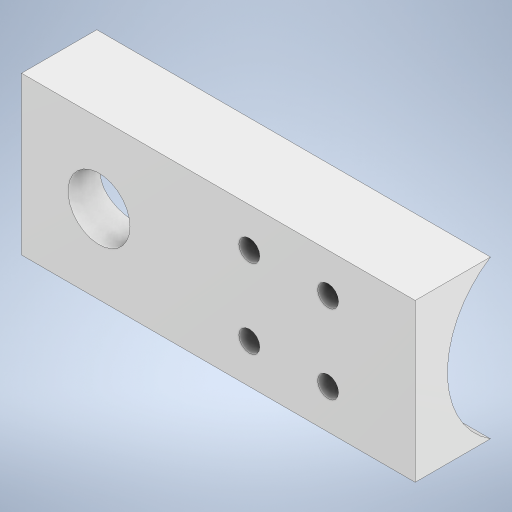
# Autodesk Inventor part: Motor Mount
Saved by Autodesk Inventor 2023 (Build 270158030, 158C)
## iProperties
Created: 2022-10-03
Part Number: Motor Mount
Material: ABS Plastic
Document SubType Name: Modeling
Designer: cjj5381
Density: 1.06 g/cm^3
Appearance: Smooth - White
Author: cjj5381
Autodesk Inventor part; units mm, degrees
ref_plane "YZ Plane" through (0, 0, 0) normal (1, 0, 0) x (0, 1, 0)
ref_plane "XZ Plane" through (0, 0, 0) normal (0, 1, 0) x (-1, 0, 0)
ref_plane "XY Plane" through (0, 0, 0) normal (0, 0, 1) x (1, 0, 0)
sketch "Sketch1" plane through (0, 0, 0) normal (1, 0, 0) x (0, 1, 0)
  arc A0 (25.4, -19.293) -> (-25.4, -19.293) centre (0, -35.56) ccw
  line L0 (0, 0) -> (0, -134.2841)
  line L1 (-25.4, 0) -> (-25.4, -19.293)
  line L2 (25.4, -19.293) -> (25.4, 0)
  line L3 (25.4, 0) -> (25.4, 5)
  line L4 (25.4, 5) -> (-25.4, 5)
  line L5 (-25.4, 5) -> (-25.4, 0)
  dimension "d0" = 60.325
  dimension "d3" = 50.8
  dimension "d38" = 5
  constraints: 12 end point, 2 perpendicular, 2 point on circle, 2 vertical, 1 centre point, 1 parallel, 1 point on line, 1 other
  measures "d0" diameter of A0
  measures "d3" distance between parallel lines of L1 L2
  measures "d38" distance from line of L0.start L4
extrude "Extrusion1" add sketch "Sketch1" along normal blind 127
sketch "Sketch4" plane through (0, 25.4, 5) normal (0, 0, 1) x (1, 0, 0)
  circle A0 centre (25, -25.4) radius 10
  line L0 (0, 0) -> (127, 0) projected
  line L1 (0, 0) -> (0, -50.8) projected
  dimension "d20" = 20
  dimension "d39" = 25.4
  dimension "d40" = 25
  constraints: 1 centre point, 1 coincident
  measures "d20" diameter of A0
  measures "d39" distance from line of point (25, -25.4) L0
  measures "d40" distance from line of point (25, -25.4) L1
extrude "Extrusion4" cut sketch "Sketch4" against normal through all
sketch "Sketch6" plane through (0, -25.4, 5) normal (0, 0, 1) x (1, 0, 0)
  line L0 (73.5, 38.1) -> (98.9, 38.1)
  line L1 (98.9, 38.1) -> (98.9, 12.7)
  line L2 (98.9, 12.7) -> (73.5, 12.7)
  line L3 (73.5, 12.7) -> (73.5, 38.1)
  line L4 (0, 0) -> (127, 0) construction
  line L5 (0, 50.8) -> (127, 50.8) projected
  line L6 (0, 50.8) -> (0, 0) projected
  point P0 (0, 25.4)
  point P1 (73.5, 25.4)
  dimension "d35" = 25.4
  dimension "d36" = 25.4
  dimension "d41" = 25.4
  dimension "d42" = 73.5
  constraints: 8 end point, 4 coincident, 2 parallel, 1 horizontal, 1 midpoint, 1 perpendicular
  measures "d35" distance of L1.end L2.end
  measures "d36" distance of L2.end L0.start
  measures "d41" distance from line of L5 point (73.5, 25.4)
  measures "d42" distance from line of L6 point (73.5, 25.4)
hole "Hole1" at (73.5, 12.7, 5) at (98.9, 12.7, 5) at (98.9, -12.7, 5) at (73.5, -12.7, 5) direction (0, 0, -1) diameter 6.756 end through all clearance for "Socket Head Cap Screw" size "1/4" standard "Ansi Unified Screw Threads"
ref_plane "Work Plane1" through (0, -25.4, -12.4625) normal (0, 0, 1) x (1, 0, 0)
sketch "Sketch7" plane through (0, -25.4, -12.4625) normal (0, 0, 1) x (1, 0, 0)
  circle A0 centre (73.5, 38.1) radius 3.378 projected
  circle A1 centre (73.5, 38.1) radius 5.08
  circle A2 centre (73.5, 12.7) radius 3.378 projected
  circle A3 centre (73.5, 12.7) radius 5.08
  circle A4 centre (98.9, 12.7) radius 3.378 projected
  circle A5 centre (98.9, 12.7) radius 5.08
  circle A6 centre (98.9, 38.1) radius 3.378 projected
  circle A7 centre (98.9, 38.1) radius 5.08
  point P0 (0, 25.4)
  dimension "d44" = 10.16
  constraints: 4 centre point, 4 coincident, 3 equal radius
  measures "d44" diameter of A1
extrude "Extrusion5" cut sketch "Sketch7" along normal blind 10 contours A0 | A1 | A2 | A3 | A4 | A5 | A6 | A7
body "Solid1"
